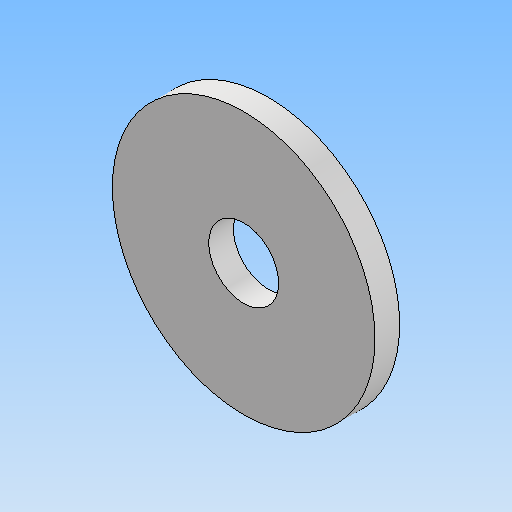
# Autodesk Inventor part: CRA-1029
Saved by Autodesk Inventor 2025.4 (Build 294407000, 407)
## iProperties
RuleStatus: InUse
Created: 2025-12-20
Part Number: CRA-1029
Material: Steel, Mild
Document SubType Name: Sheet Metal
Designer: josh
Mass: 70.4128 g
Surface Area: 47.2908 cm^2
Volume: 8.96979 cm^3
Density: 7.85 g/cm^3
Flat Pattern Width: 5.08 cm
Flat Pattern Length: 5.08 cm
Flat Pattern Area: 25.8064 cm^2
Sheet Metal Rule: Mild Steel .188
Sheet Metal Width: 2.000 in
Sheet Metal Length: 2.000 in
Sheet Metal Area: 4.000 in^2
Appearance: Default
Description: 2" OD X 1/2"ID FENDER WASHER
AfterDocOpen0: PartNumber
Flat pattern length: =<Sheet Metal Length>
Flat pattern width: =<Sheet Metal Width>
Thickness: 0.188 in
Qty: 1
Flat Length: 2.0
Flat Width: 2.0
Part Area: 4.0
Author: josh
Autodesk Inventor part; units mm, degrees
ref_plane "YZ Plane" through (0, 0, 0) normal (1, 0, 0) x (0, 1, 0)
ref_plane "XZ Plane" through (0, 0, 0) normal (0, 1, 0) x (-1, 0, 0)
ref_plane "XY Plane" through (0, 0, 0) normal (0, 0, 1) x (1, 0, 0)
sketch "Sketch12" plane through (0, 0, 0) normal (0, 0, 1) x (1, 0, 0)
  circle A0 centre (0, 0) radius 25.4
  circle A1 centre (0, 0) radius 6.7564
  dimension "d107" = 50.8
  dimension "d108" = 13.5128
  measures "d107" diameter of A0
  measures "d108" diameter of A1
extrude "Plate4" add sketch "Sketch12" along normal blind 4.7625
equation "\"d109\" = Thickness"
equation "\"BendRadius\" = Thickness"
equation "\"BendReliefWidth\" = Thickness"
equation "\"BendReliefDepth\" = 0.5 * Thickness"
equation "\"CornerReliefSize\" = 4 * Thickness"
equation "\"MinimumRemnant\" = 2 * Thickness"
equation "\"TransitionRadius\" = BendRadius"
equation "\"JacobiRadiusSize\" = BendRadius"
equation "\"GapSize\" = Thickness"
equation "\"Thickness\" = 4.7625"
body "Solid3"
